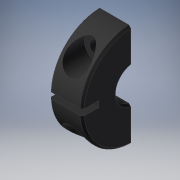
# Autodesk Inventor part: C-SCNPAW8-8_1
Saved by Autodesk Inventor 2019 (Build 230136000, 136)
## iProperties
Created: 2023-10-02
Part Number: C-SCNPAW8-8_1
Material: Generic
Catalog Web Link: www.cadenas.de
Description: C-SCNPAW_1-Economy Shaft Collars - Split
Vendor: MISUMI
Document SubType Name: Modeling
Designer: psAdmin
Manufacturer: MISUMI
Mass: 1.27485 g
Surface Area: 11.5524 cm^2
Volume: 1.27485 cm^3
Density: 1 g/cm^3
Appearance: PSOLRGB-175-175-175
Category: PARTsolutions
Company: MISUMI
Title: C-SCNPAW8-8
Author: Cadenas PARTsolutions
Comments: Economy Shaft Collars - Split
PSOL_IDENT_0: {$CADENAS_DATA/23d-libs/misumi/metric/03_set_collars/c_scnpaw/c_scnpaw_1.prj},170 {VTYP=3D},{NB=C-SC
PSOL_IDENT_1: NPAW8-8_1},{LINA=C-SCNPAW8-8},{NN=C-SCNPAW_1},{DATE=12.09.2022 02:00:34},{GEOMDATE=08.03.2021 11:40:
PSOL_IDENT_2: 51},{VERSION=},{LINEID=20},{WBVAR=B},{WBNUMERIC=B}  {NB=C-SCNPAW8-8_1},{LINA=C-SCNPAW8-8},{KT=DUMMY}
PSOL_IDENT_3: ,{PN=C-SCNPAW8-8},{D=8},{B=8},{BALG=8,10},{D1=25},{M1=M3},{M=3},{DD=3.4},{H=6.0},{W=1.5},{X=8.0},{Y=
PSOL_IDENT_4: 5},{C=0.5},{L=10},{HH=4.0}
NB: C-SCNPAW8-8_1
NN: C-SCNPAW_1
NT: Economy Shaft Collars - Split
NBSYN: $PN._1
LINA: C-SCNPAW8-8
CATALOG: Misumi
PN: C-SCNPAW8-8
D: 8
B: 8
D1: 25
M1: M3
DD: 3.4
H: 6
W: 1.5
X: 8
Y: 5
SUPPLIER: MISUMI
ARTICLENO: C-SCNPAW8-8_1
BOMINFO: C-SCNPAW8-8
CREATOR: CADENAS GmbH
Autodesk Inventor part; units mm, degrees
sketch "_____1" plane through (0, 0, 0) normal (0, 0, 1) x (1, 0, 0)
  line L0 (50, 0) -> (-50, 0)
  line L1 (-4, 12) -> (-4, 4.5)
  line L2 (-4, 4.5) -> (-3.5, 4)
  line L3 (-3.5, 4) -> (3.5, 4)
  line L4 (3.5, 4) -> (4, 4.5)
  line L5 (4, 4.5) -> (4, 12)
  line L6 (4, 12) -> (3.5, 12.5)
  line L7 (3.5, 12.5) -> (-3.5, 12.5)
  line L8 (-3.5, 12.5) -> (-4, 12)
  constraints: 18 end point
revolve "Revolution1" add sketch "_____1" angle 180 about axis through (50, 0, 0) along (1, 0, 0)
sketch "_____2" plane through (0, 0, 0) normal (1, 0, 0) x (0, 0, -1)
  line L0 (-0.75, -25) -> (0.75, -25)
  line L1 (0.75, -25) -> (0.75, 25)
  line L2 (0.75, 25) -> (-0.75, 25)
  line L3 (-0.75, 25) -> (-0.75, -25)
  constraints: 8 end point
extrude "Extrusion1" cut sketch "_____2" along normal mid plane 16
sketch "_____3" plane through (0, 0, 0) normal (1, 0, 0) x (0, 0, -1)
  line L0 (0, 8) -> (-17.5, 8)
  line L1 (-17.5, 8) -> (-17.5, 11)
  line L2 (-17.5, 11) -> (-5, 11)
  line L3 (-5, 11) -> (-5, 9.7)
  line L4 (-5, 9.7) -> (0, 9.7)
  line L5 (0, 9.7) -> (0, 8)
  line L6 (0, 8) -> (-17.5, 8)
  constraints: 14 end point
revolve "Revolution2" cut sketch "_____3" angle 360 about axis through (0, 8, 0) along (0, 0, -1)
pattern_linear "Rectangular Pattern1" count 2 spacing 16 along (0, -1, 0) of "Revolution2"
sketch "_____5" plane through (0, 0, 0) normal (1, 0, 0) x (0, 0, -1)
  line L0 (-12.5, -0.75) -> (-8.5, -0.75)
  line L1 (-8.5, -0.75) -> (-8.5, 0.75)
  line L2 (-8.5, 0.75) -> (-12.5, 0.75)
  line L3 (-12.5, 0.75) -> (-12.5, -0.75)
  constraints: 8 end point
extrude "Extrusion2" cut sketch "_____5" along normal mid plane 16
ref_plane "to_body_XY" through (0, 0, 0) normal (0, 0, -1) x (1, 0, 0)
ref_plane "to_body_YZ" through (0, 0, 0) normal (1, 0, 0) x (0, -1, 0)
ref_plane "to_body_ZX" through (0, 0, 0) normal (0, -1, 0) x (0, 0, -1)
ref_plane "to_bolt_1_XY" through (0, 8, 5) normal (0, 0, 1) x (1, 0, 0)
ref_plane "to_bolt_1_YZ" through (0, 8, 5) normal (1, 0, 0) x (0, 1, 0)
ref_plane "to_bolt_1_ZX" through (0, 8, 5) normal (0, 1, 0) x (0, 0, 1)
ref_plane "to_bolt_2_XY" through (0, -8, 5) normal (0, 0, 1) x (1, 0, 0)
ref_plane "to_bolt_2_YZ" through (0, -8, 5) normal (1, 0, 0) x (0, 1, 0)
ref_plane "to_bolt_2_ZX" through (0, -8, 5) normal (0, 1, 0) x (0, 0, 1)
body "Solid1"
